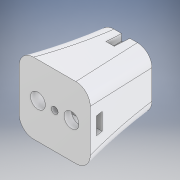
# Autodesk Inventor part: AA016b
Saved by Autodesk Inventor 2017 SP1 (Build 210196100, 196)
## iProperties
Created: 2017-09-29
Part Number: AA016b
Material: ABS Plastic
Document SubType Name: Modeling
Designer: Zach
Density: 1.06 g/cm^3
Appearance: CR White
Author: Zach
Autodesk Inventor part; units mm, degrees
ref_plane "XZ Plane" through (0, 0, 0) normal (0, 1, 0) x (-1, 0, 0)
ref_plane "XY Plane" through (0, 0, 0) normal (0, 0, 1) x (1, 0, 0)
sketch "Sketch1" plane through (0, 0, 0) normal (0, 0, 1) x (1, 0, 0)
  line L0 (0, 0) -> (70, 0)
  line L1 (70, 0) -> (70, 77.5)
  line L2 (70, 77.5) -> (0, 77.5)
  line L3 (0, 77.5) -> (0, 0)
  dimension "d0" = 70
  dimension "d1" = 77.5
  constraints: 8 end point, 2 parallel, 1 horizontal, 1 perpendicular
  measures "d0" distance of L2.end L1.end
  measures "d1" distance of L1.end L0.end
extrude "Extrusion1" add sketch "Sketch1" along normal blind 95
sketch "Sketch3" plane through (0, 0, 95) normal (0, 0, 1) x (1, 0, 0)
  line L0 (0, 0) -> (70, 0) projected
  line L1 (70, 77.5) -> (0, 77.5) projected
  line L2 (70, 0) -> (35, 0)
  line L3 (35, 0) -> (35, 77.5)
  line L4 (35, 77.5) -> (70, 77.5)
  line L5 (70, 77.5) -> (70, 0)
  constraints: 8 end point, 2 parallel, 1 horizontal, 1 midpoint, 1 perpendicular
extrude "Extrusion3" cut sketch "Sketch3" against normal through all
sketch "Sketch4" plane through (0, 77.5, 95) normal (0, 1, 0) x (1, 0, 0)
  line L0 (0, 95) -> (0, 0) projected
  line L1 (0, 0) -> (-12.5, 0)
  line L2 (35, 95) -> (0, 95) projected
  arc A0 (-12.5, 0) -> (0, 95) centre (-1145.4326, 197.3924) ccw
  line L3 (-12.5, -10) -> (35, -10) construction
  dimension "d9" = 1150
  dimension "d54" = 47.5
  dimension "d55" = 10
  constraints: 4 end point, 2 horizontal, 2 point on circle, 2 vertical alignment, 1 centre point
  measures "d9" radius of A0
  measures "d54" distance of L3.start L3.end
  measures "d55" distance between parallel lines of L1 L3
extrude "Extrusion4" add sketch "Sketch4" against normal blind 77.5
sketch "Sketch5" plane through (35, 0, 95) normal (1, 0, 0) x (0, 0, -1)
  line L0 (0, 77.5) -> (0, 86.25)
  line L1 (0, 0) -> (0, -8.75)
  line L2 (0, 0) -> (0, 77.5) projected
  line L3 (95, 77.5) -> (95, 0) projected
  arc A0 (0, 86.25) -> (95, 77.5) centre (152.8838, 1226.0423) ccw
  arc A1 (95, 0) -> (0, -8.75) centre (152.8838, -1148.5423) ccw
  line L4 (0, 77.5) -> (95, 77.5) projected
  line L5 (95, 0) -> (0, 0) projected
  line L6 (-10, 86.25) -> (-10, -8.75) construction
  point P0 (-10, 38.75)
  point P1 (0, 38.75)
  dimension "d14" = 1150
  dimension "d15" = 1150
  dimension "d52" = 10
  dimension "d53" = 95
  constraints: 6 end point, 4 point on circle, 3 horizontal alignment, 3 vertical, 2 centre point, 2 midpoint
  measures "d14" radius of A0
  measures "d15" radius of A1
  measures "d52" distance between parallel lines of L2 L6
  measures "d53" distance of L6.start L6.end
extrude "Extrusion5" add sketch "Sketch5" against normal blind 55 contours L0 A0 L4 | L5 A1 L1
sketch "Sketch6" plane through (-20, 0, 0) normal (0, 1, 0) x (1, 0, 0)
  line L0 (20, 0) -> (0, 0) projected
  line L1 (0, -95) -> (0, 0) projected
  arc A0 (7.5, -95) -> (20, 0) centre (-1125.4326, 102.3924) ccw projected
  line L2 (7.5, -95) -> (0, -95) projected
extrude "Extrusion6" cut sketch "Sketch6" along normal through all both and the other way through all
fillet "Fillet3" radius 19.35 2 edges at (-5.299, 80.9203, 47.9253) (-5.299, -3.4203, 47.9253)
sketch "Sketch56" plane through (0, 0, 95) normal (0, 0, 1) x (1, 0, 0)
  line L0 (35, 77.5) -> (35, 0) projected
  circle A0 centre (35, 38.75) radius 4.5
  point P0 (0, 0)
  dimension "d183" = 9
  constraints: 1 centre point, 1 midpoint
  measures "d183" diameter of A0
extrude "Extrusion46" cut sketch "Sketch56" against normal through all
ref_plane "Work Plane10" through (0, 0, 85) normal (0, 0, 1) x (1, 0, 0)
sketch "Sketch57" plane through (0, 0, 85) normal (0, 0, 1) x (1, 0, 0)
  arc A0 (35, 43.25) -> (35, 34.25) centre (35, 38.75) ccw projected
  circle A1 centre (35, 38.75) radius 11.5
  point P0 (0, 0)
  dimension "d187" = 23
  constraints: 1 centre point, 1 coincident
  measures "d187" diameter of A1
extrude "Extrusion47" cut sketch "Sketch57" against normal blind 9
ref_plane "Work Plane11" through (0, 0, 30) normal (0, 0, -1) x (-1, 0, 0)
sketch "Sketch58" plane through (0, 0, 30) normal (0, 0, -1) x (-1, 0, 0)
  arc A0 (-35, 34.25) -> (-35, 43.25) centre (-35, 38.75) ccw projected
  line L0 (-35, 50.25) -> (-35, 43.25) projected
  arc A1 (-35, 27.25) -> (-35, 50.25) centre (-35, 38.75) ccw projected
  line L1 (-35, 34.25) -> (-35, 27.25) projected
  arc A2 (-35, 34.25) -> (-35, 43.25) centre (-35, 38.75) ccw projected
  point P0 (0, 0)
extrude "Extrusion48" cut sketch "Sketch58" against normal blind 9
mirror "Mirror1" about plane through (35, 0, 95) normal (1, 0, 0)
sketch "Sketch59" plane through (35, 38.75, 76) normal (0, 0, 1) x (1, 0, 0)
  circle A0 centre (0, 0) radius 4.5 projected
  circle A1 centre (0, 0) radius 11.5 construction
  circle A2 centre (0, 0) radius 11.5 construction
  line L0 (0, 11.5) -> (50, 11.5)
  line L1 (0, -11.5) -> (50, -11.5)
  line L2 (50, -11.5) -> (50, 11.5)
  line L3 (0, -11.5) -> (0, 11.5)
  point P0 (-35, -38.75)
  dimension "d193" = 50
  constraints: 8 end point, 4 point on circle, 3 tangent, 2 vertical, 2 vertical alignment, 1 horizontal
  measures "d193" distance from line of A0.centre L2
extrude "Extrusion49" cut sketch "Sketch59" along normal blind 9 contours A0 L3 | A0 L3 L0 L2 L1 picked at (0.6508, -1.3515)
sketch "Sketch60" plane through (35, 38.75, 39) normal (0, 0, -1) x (-1, 0, 0)
  circle A0 centre (0, 0) radius 11.5 construction
  circle A1 centre (0, 0) radius 4.5 projected
  circle A2 centre (0, 0) radius 11.5 projected
  line L0 (0, 11.5) -> (47.5, 11.5)
  line L1 (0, -11.5) -> (47.5, -11.5)
  line L2 (47.5, -11.5) -> (47.5, 11.5)
  line L3 (0, -11.5) -> (0, 11.5)
  line L4 (47.5, 28.4225) -> (47.5, -28.4225) projected
  point P0 (35, -38.75)
  point P1 (47.5, 0)
  constraints: 8 end point, 4 point on circle, 3 tangent, 2 horizontal, 2 midpoint, 1 perpendicular, 1 point on line
extrude "Extrusion50" cut sketch "Sketch60" along normal blind 9 contours A1 L3 | A1 L3 A2 | L0 L2 L1 A2 picked at (0.6508, -1.3515) picked at (9.0329, -1.1868)
sketch "Sketch61" plane through (0, 0, 95) normal (0, 0, 1) x (1, 0, 0)
  circle A0 centre (57.5, 38.75) radius 2.5
  circle A1 centre (12.5, 38.75) radius 2.5
  circle A2 centre (35, 38.75) radius 4.5 construction
  line L0 (57.5, 38.75) -> (12.5, 38.75) construction
  point P0 (0, 0)
  dimension "d198" = 5
  dimension "d199" = 5
  dimension "d200" = 45
  constraints: 2 centre point, 2 end point, 1 coincident, 1 horizontal, 1 midpoint
  measures "d198" diameter of A0
  measures "d199" diameter of A1
  measures "d200" distance of L0.start L0.end
extrude "Extrusion51" cut sketch "Sketch61" against normal through all
ref_plane "Work Plane12" through (0, 0, 5) normal (0, 0, -1) x (-1, 0, 0)
sketch "Sketch63" plane through (0, 0, 5) normal (0, 0, -1) x (-1, 0, 0)
  circle A0 centre (-12.5, 38.75) radius 2.5 projected
  circle A1 centre (-57.5, 38.75) radius 2.5 projected
  circle A2 centre (-12.5, 38.75) radius 10
  circle A3 centre (-57.5, 38.75) radius 10
  point P0 (0, 0)
  dimension "d205" = 20
  dimension "d206" = 20
  constraints: 2 centre point, 2 coincident
  measures "d205" diameter of A2
  measures "d206" diameter of A3
extrude "Extrusion52" cut sketch "Sketch63" against normal through all
sketch "Sketch65" plane through (0, 0, 0) normal (0, 0, -1) x (-1, 0, 0)
  circle A0 centre (-35, 38.75) radius 4.5 projected
  circle A1 centre (-35, 38.75) radius 12.5
  point P0 (0, 0)
  dimension "d209" = 25
  constraints: 1 centre point, 1 coincident
  measures "d209" diameter of A1
extrude "Extrusion53" cut sketch "Sketch65" against normal blind 25
ref_plane "Work Plane13" through (35, 77.5, 0) normal (1, 0, 0) x (0, 1, 0)
sketch "Sketch66" plane through (35, 77.5, 0) normal (1, 0, 0) x (0, 1, 0)
  line L0 (0, 0) -> (-9, 0)
  line L1 (-9, 0) -> (-9, 21)
  line L2 (-9, 21) -> (1.251, 21)
  arc A0 (1.251, 21) -> (0, 0) centre (1148.5423, -57.8838) ccw
  line L3 (-19.2875, 0) -> (-58.2125, 0) projected
  line L4 (-38.75, 0) -> (-38.75, 95)
  line L5 (-77.5, 0) -> (-68.5, 0)
  line L6 (-68.5, 0) -> (-68.5, 21)
  line L7 (-68.5, 21) -> (-78.751, 21)
  arc A1 (-77.5, 0) -> (-78.751, 21) centre (-1226.0423, -57.8838) ccw
  point P0 (-77.5, 0)
  dimension "d212" = 9
  dimension "d213" = 21
  dimension "d214" = 1150
  constraints: 14 end point, 5 symmetric about line, 4 point on circle, 2 centre point, 2 perpendicular, 1 horizontal, 1 midpoint, 1 vertical, 3 other
  measures "d212" distance of L0.start L0.end
  measures "d213" distance of L0.end L1.end
  measures "d214" radius of A0
extrude "Extrusion54" cut sketch "Sketch66" along normal mid plane 11
sketch "Sketch67" plane through (29.5, 68.5, 0) normal (0, 1, 0) x (1, 0, 0)
  circle A0 centre (5.5, -10) radius 2.5
  line L0 (0, 0) -> (11, 0) projected
  point P0 (-29.5, 0)
  point P1 (5.5, 0)
  dimension "d217" = 5
  dimension "d218" = 10
  constraints: 1 centre point, 1 midpoint, 1 vertical alignment
  measures "d217" diameter of A0
  measures "d218" distance from line of L0 A0.centre
extrude "Extrusion55" cut sketch "Sketch67" against normal through all
body "Solid1"
